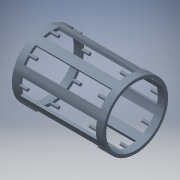
# Autodesk Inventor part: BearingHolderCJE
Saved by Autodesk Inventor 2018 (Build 220112000, 112)
## iProperties
Created: 2018-02-03
Part Number: BearingHolderCJE
Material: Titanium
Document SubType Name: Modeling
Designer: textboox5
Density: 4.51 g/cm^3
Appearance: Steel Blue
Author: textboox5
Autodesk Inventor part; units mm, degrees
ref_plane "YZ Plane" through (0, 0, 0) normal (1, 0, 0) x (0, 1, 0)
ref_plane "XZ Plane" through (0, 0, 0) normal (0, 1, 0) x (-1, 0, 0)
ref_plane "XY Plane" through (0, 0, 0) normal (0, 0, 1) x (1, 0, 0)
sketch "Sketch1" plane through (0, 0, 0) normal (0, 0, 1) x (1, 0, 0)
  line L0 (-1574.8, 0) -> (1574.8, 0) construction
  line L1 (-1574.8, -1066.8) -> (1574.8, -1066.8) construction
  line L2 (0, 0) -> (0, -1066.8) construction
  line L3 (-1574.8, -1016) -> (-1574.8, -1066.8)
  line L4 (-1574.8, -1117.6) -> (1574.8, -1117.6)
  line L5 (1574.8, -1117.6) -> (1574.8, -1066.8)
  line L6 (1574.8, -1066.8) -> (1574.8, -1016)
  line L7 (1574.8, -1016) -> (-1574.8, -1016)
  line L8 (-1574.8, -1066.8) -> (-1574.8, -1117.6)
  dimension "d4" = 101.6
  dimension "d18" = 1066.8
  dimension "d19" = 3149.6
  constraints: 18 end point, 4 perpendicular, 3 point on line, 2 horizontal, 2 midpoint, 2 parallel, 1 vertical, 1 other
  measures "d4" distance between parallel lines of L4 L7
  measures "d18" distance between parallel lines of L1 L0
  measures "d19" distance of L4.start L4.end
revolve "Revolution1" add sketch "Sketch1" angle 360 about axis through (-1574.8, 0, 0) along (1, 0, 0)
sketch "Sketch2" plane through (0, 0, 0) normal (0, 0, 1) x (1, 0, 0)
  line L0 (1320.8, -1016) -> (1320.8, -1117.6)
  line L1 (-1320.8, -1016) -> (-1320.8, -1117.6)
  line L2 (0, -1016) -> (0, 0) construction
  line L3 (1320.8, -1016) -> (-1320.8, -1016)
  line L4 (-1320.8, -1117.6) -> (1320.8, -1117.6)
  line L5 (-2205.8938, 0) -> (2205.8938, 0) projected
  line L6 (-1574.8, -1117.6) -> (1574.8, -1117.6) construction
  line L7 (1574.8, -1016) -> (-1574.8, -1016) construction
  point P0 (1574.8, 1016)
  dimension "d16" = 254
  constraints: 10 end point, 3 vertical, 2 collinear, 2 perpendicular, 1 midpoint, 1 other
  measures "d16" distance of L6.end L0.end
revolve "Revolution2" cut sketch "Sketch2" angle 45 mid plane about axis through (-10, 0, 0) along (1, 0, 0)
sketch "Sketch3" plane through (1320.8, 0, 0) normal (-1, 0, 0) x (0, 0, 1)
  circle A0 centre (0, -1066.8) radius 50.8
  circle A1 centre (0, 0) radius 1016 construction
  circle A2 centre (0, 0) radius 1117.6 construction
  line L0 (0, -1066.8) -> (0, 0) construction
  constraints: 2 end point, 2 tangent, 1 centre point, 1 vertical
extrude "Extrusion1" add sketch "Sketch3" along normal blind 254
mirror "Mirror1" about plane through (0, 0, 0) normal (1, 0, 0) of "Extrusion1"
pattern_circular "Circular Pattern1" count 6 over 360 about axis through (-10, 0, 0) along (1, 0, 0) of "Extrusion1", "Mirror1", "Revolution2"
body "Solid1"
